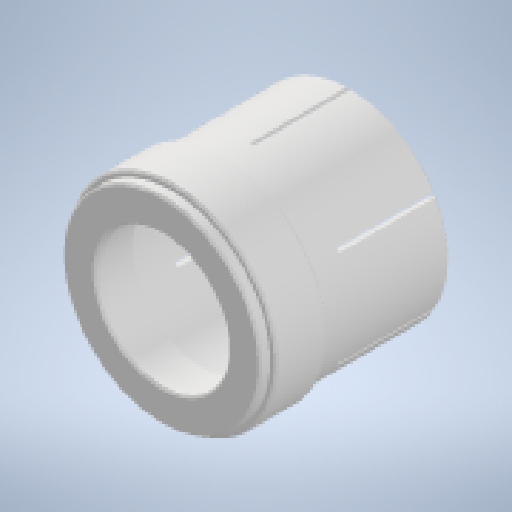
# Autodesk Inventor part: Nikon50mm-barebone-mount
Saved by Autodesk Inventor 2024 (Build 280153000, 153)
## iProperties
Created: 2026-01-13
Part Number: Nikon50mm-barebone-mount
Material: Generic
Document SubType Name: Modeling
Designer: nvladi
Density: 1 g/cm^3
Appearance: Default
Author: nvladi
Autodesk Inventor part; units mm, degrees
ref_plane "YZ Plane" through (0, 0, 0) normal (1, 0, 0) x (0, 1, 0)
ref_plane "XZ Plane" through (0, 0, 0) normal (0, 1, 0) x (-1, 0, 0)
ref_plane "XY Plane" through (0, 0, 0) normal (0, 0, 1) x (1, 0, 0)
sketch "Sketch2" plane through (0, 0, 0) normal (1, 0, 0) x (0, 1, 0)
  line L0 (17.05, -2) -> (17.05, -10)
  line L1 (17.05, -10) -> (21.3, -10)
  line L2 (21.3, -10) -> (21.3, -46)
  line L3 (21.3, -46) -> (24, -46)
  line L4 (24, -46) -> (24, -15)
  line L5 (24, -15) -> (25.4, -15)
  line L6 (25.4, -15) -> (25.4, -2.5)
  line L7 (25.4, 0) -> (17.05, 0)
  line L8 (0, 0) -> (0, -55.6888)
  line L9 (17.05, 0) -> (16.15, 0)
  line L10 (16.15, 0) -> (16.15, -2)
  line L11 (16.15, -2) -> (17.05, -2)
  line L12 (17.05, -2) -> (17.05, 0)
  line L13 (25.4, 0) -> (24, 0)
  line L14 (24, 0) -> (24, -2.5)
  line L15 (24, -2.5) -> (25.4, -2.5)
  line L16 (25.4, -2.5) -> (25.4, -2)
  point P0 (24.7, -15)
  dimension "d0" = 10
  dimension "d1" = 36
  dimension "d2" = 17.05
  dimension "d3" = 21.3
  dimension "d4" = 25.4
  dimension "d5" = 24
  dimension "d6" = 15
  dimension "d7" = 2
  dimension "d8" = 0.9
  dimension "d14" = 1.4
  dimension "d15" = 2.5
  constraints: 34 end point, 9 perpendicular, 4 parallel, 3 horizontal, 2 vertical, 1 midpoint, 1 point on line
  measures "d0" distance of L7.end L0.end
  measures "d1" distance of L1.end L2.end
  measures "d2" distance between parallel lines of L8 L0
  measures "d3" distance between parallel lines of L8 L2
  measures "d4" distance between parallel lines of L8 L6
  measures "d5" distance between parallel lines of L8 L4
  measures "d6" distance from line of point (24.7, -15) L7
  measures "d7" distance of L10.end L9.end
  measures "d8" distance between parallel lines of L10 L0
  measures "d14" distance of L6.end L14.end
  measures "d15" distance of L14.end L13.end
revolve "Revolution2" add sketch "Sketch2" angle 360 about axis through (0, 0, 0) along (0, 0, -1)
chamfer "Chamfer1" distance 0.5 angle 45 4 edges at (0, -25.4, -15) (0, -16.15, 0) (0, -24, -46) (0, -21.3, -46)
chamfer "Chamfer2" distance 0.5 angle 45 2 edges at (0, -24, 0) (0, -25.4, -2.5)
sketch "Sketch4" plane through (0, 0, -46) normal (0, 0, -1) x (-1, 0, 0)
  line L0 (0.5, 17.8994) -> (-0.5, 17.8994)
  line L1 (-0.5, 17.8994) -> (-0.5, 25.7006)
  line L2 (-0.5, 25.7006) -> (0.5, 25.7006)
  line L3 (0.5, 25.7006) -> (0.5, 17.8994)
  circle A0 centre (0, 0) radius 21.8 projected
  line L4 (0.5, 17.8994) -> (-0.5, 25.7006) construction
  line L5 (-0.5, 17.8994) -> (0.5, 25.7006) construction
  point P0 (0, 21.8)
  dimension "d19" = 1
  constraints: 12 end point, 2 midpoint, 2 parallel, 1 horizontal, 1 perpendicular, 1 vertical alignment, 1 other
  measures "d19" distance of L1.end L2.end
extrude "Extrusion1" cut sketch "Sketch4" against normal blind 24 contours L0 L1 A0 L3 | A0 L1 L2 L3 picked at (0.0556, 19.1994)
pattern_circular "Circular Pattern1" count 6 over 360 about axis through (0, 0, -10) along (0, 0, 1) of "Extrusion1"
fillet "Fillet1" radius 0.5 2 edges at (-0.5, 22.6445, -22) (0.5, 22.6445, -22)
pattern_circular "Circular Pattern2" count 6 over 360 about axis through (0, 0, -10) along (0, 0, 1) of "Fillet1"
body "Solid1"
